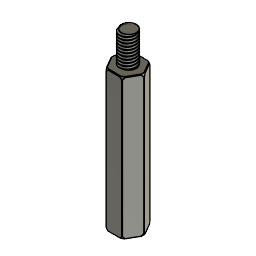
M3 X 25mm Male to Female Brass Spacer (Autodesk Fusion 360 design; units mm, degrees)
Autodesk Fusion 360 part; units mm, degrees
sketch "Sketch1" plane through (0, 0, 0) normal (0, 0, 1) x (1, 0, 0)
  line L0 (-1.4434, 2.5) -> (-2.8868, 0)
  line L1 (-2.8868, 0) -> (-1.4434, -2.5)
  line L2 (-1.4434, -2.5) -> (1.4434, -2.5)
  line L3 (1.4434, -2.5) -> (2.8868, 0)
  line L4 (2.8868, 0) -> (1.4434, 2.5)
  line L5 (1.4434, 2.5) -> (-1.4434, 2.5)
  circle A0 centre (0, 0) radius 1.5
  dimension "d2" = 3
  constraint coincident A0.centre origin
  measures "d2" diameter of A0
extrude "Extrude1" add sketch "Sketch1" along normal blind 25
extrude "Extrude2" add sketch "Sketch1" along normal blind 22.5 from surface at 8 contours A0
thread "Thread1" "ISO Metric profile 3.0 M3x0.5 M3x0.5 6g" major diameter 2.927 minor diameter 2.3555 pitch 0.5 angle 60 modelled right hand crest width 0.0713 on face at (1.4925, -0.1494, 26.8333) crest through (1.4635, 0, 24.875)
thread "Thread2" "ISO Metric profile 3.0 M3x0.5 M3x0.5 6H" major diameter 3.086 minor diameter 2.529 pitch 0.5 angle 60 modelled right hand crest width 0.1368 on face at (1.4925, -0.1494, 2.6667) crest through (1.2645, 0, 0.125)
sketch "Sketch2" plane through (-2.1651, -1.25, 0) normal (-0.866025, -0.5, 0) x (0.5, -0.866025, 0)
  line L0 (-1.4434, 0) -> (1.4434, 0)
  line L1 (1.4434, 0) -> (1.4434, 25)
  line L2 (1.4434, 25) -> (-1.4434, 25)
  line L3 (-1.4434, 25) -> (-1.4434, 0)
  line L4 (-1.4434, 0) -> (-1.4434, 0.5)
  line L5 (-1.4434, 25) -> (-1.4434, 24.5)
  dimension "d12" = 0.5
  dimension "d13" = 0.5
  constraint coincident L0.start L3.end
  constraint perpendicular L0 L4
  constraint coincident L2.end L3.start
  constraint perpendicular L2 L5
  measures "d12" distance of L0.start L4.end
  measures "d13" distance of L2.end L5.end
sketch "Sketch3" plane through (0, 0, 25) normal (0, 0, 1) x (-1, 0, 0)
  arc A0 (-0.634, -1.319) -> (0.634, -1.319) centre (0, 0) ccw
  spline S0 degree 3 poles (-0.634, -1.319) (-0.7449, -1.2523) (-0.8463, -1.1711) (-1.0222, -0.9858) (-1.0965, -0.8832) (-1.239, -0.6161) (-1.2915, -0.4458) (-1.3263, -0.1013) (-1.3109, 0.0692) (-1.2163, 0.3878) (-1.1406, 0.5335) (-0.941, 0.7816) (-0.821, 0.8831) (-0.6847, 0.9583) knots -0.275362 -0.275362 -0.275362 -0.275362 -0.236706 -0.236706 -0.199015 -0.199015 -0.146206 -0.146206 -0.095434 -0.095434 -0.046698 -0.046698 0 0 0 0
  arc A1 (0.6847, 0.9583) -> (-0.6847, 0.9583) centre (0, 0) ccw
  spline S1 degree 3 poles (0.6847, 0.9583) (0.7781, 0.9068) (0.864, 0.8428) (1.019, 0.6916) (1.0868, 0.6046) (1.2259, 0.367) (1.2801, 0.209) (1.3272, -0.1257) (1.317, -0.2994) (1.2301, -0.6403) (1.1516, -0.8035) (0.9334, -1.097) (0.7937, -1.2229) (0.634, -1.319) knots -0.276632 -0.276632 -0.276632 -0.276632 -0.244511 -0.244511 -0.211432 -0.211432 -0.161639 -0.161639 -0.109803 -0.109803 -0.055923 -0.055923 0 0 0 0
  line L0 (-1.4434, -2.5) -> (1.4434, -2.5)
  line L1 (1.4434, -2.5) -> (2.8868, 0)
  line L2 (2.8868, 0) -> (1.4434, 2.5)
  line L3 (1.4434, 2.5) -> (-1.4434, 2.5)
  line L4 (-1.4434, 2.5) -> (-2.8868, 0)
  line L5 (-2.8868, 0) -> (-1.4434, -2.5)
  line L6 (2.8868, 0) -> (2.6368, 0.433)
  line L7 (2.8868, 0) -> (2.6368, -0.433)
  dimension "d14" = 0.5
  dimension "d15" = 0.5
  constraint coincident L1.end L2.start
  constraint parallel L2 L6
  constraint parallel L1 L7
  measures "d14" distance of L1.end L6.end
  measures "d15" distance of L1.end L7.end
sketch "Sketch4" plane through (0, 0, 0) normal (0, 0, -1) x (1, 0, 0)
  spline S0 degree 3 poles (-0.3985, -1.4906) (-0.5834, -1.4231) (-0.7535, -1.3207) (-1.0389, -1.0601) (-1.1532, -0.9065) (-1.3124, -0.5696) (-1.3581, -0.3908) (-1.3767, -0.0326) (-1.352, 0.1432) (-1.259, 0.4082) (-1.2125, 0.5028) (-1.099, 0.6765) (-1.033, 0.7553) (-0.9581, 0.8252) knots 0 0 0 0 0.059039 0.059039 0.116033 0.116033 0.170983 0.170983 0.223888 0.223888 0.255505 0.255505 0.286347 0.286347 0.286347 0.286347
  arc A0 (0.9581, 0.8252) -> (-0.9581, 0.8252) centre (0, 0) ccw
  spline S1 degree 3 poles (0.9581, 0.8252) (1.0802, 0.7112) (1.1784, 0.574) (1.3207, 0.264) (1.3611, 0.093) (1.3757, -0.2618) (1.3471, -0.4423) (1.2212, -0.7891) (1.1226, -0.9512) (0.9156, -1.1792) (0.8244, -1.2577) (0.6232, -1.3929) (0.5136, -1.4486) (0.3985, -1.4906) knots 0 0 0 0 0.050111 0.050111 0.102261 0.102261 0.15645 0.15645 0.212677 0.212677 0.24852 0.24852 0.285143 0.285143 0.285143 0.285143
  arc A1 (-0.3985, -1.4906) -> (0.3985, -1.4906) centre (0, 0) ccw
  line L0 (-1.4434, -2.5) -> (1.4434, -2.5)
  line L1 (1.4434, -2.5) -> (2.8868, 0)
  line L2 (2.8868, 0) -> (1.4434, 2.5)
  line L3 (1.4434, 2.5) -> (-1.4434, 2.5)
  line L4 (-1.4434, 2.5) -> (-2.8868, 0)
  line L5 (-2.8868, 0) -> (-1.4434, -2.5)
  line L6 (-2.8868, 0) -> (-2.6368, 0.433)
  line L7 (-2.8868, 0) -> (-2.6368, -0.433)
  dimension "d16" = 0.5
  dimension "d17" = 0.5
  constraint coincident L4.end L5.start
  constraint parallel L4 L6
  constraint parallel L5 L7
  measures "d16" distance of L4.end L6.end
  measures "d17" distance of L4.end L7.end
ref_plane "WorkPlane1" through (-2.6368, 0.433, 25) normal (0.894427, 0, -0.447214) x (-0.447214, 0, -0.894427)
ref_plane "WorkPlane2" through (-2.6368, 0.433, 0) normal (0.894427, 0, 0.447214) x (0.447214, 0, -0.894427)
sketch "Sketch5" plane through (-2.1094, 0, -1.0547) normal (0.894427, 0, 0.447214) x (0.447214, 0, -0.894427)
  line L0 (-1.8, -0.5) -> (-1.1, -0.5)
  line L1 (-1.1, -0.5) -> (-1.1, 0.5)
  line L2 (-1.1, 0.5) -> (-1.8, 0.5)
  line L3 (-1.8, 0.5) -> (-1.8, -0.5)
  constraint horizontal L0
  constraint vertical L1
  constraint horizontal L2
  constraint vertical L3
extrude "Extrude3" cut sketch "Sketch5" against normal blind 5
sketch "Sketch6" plane through (-12.1094, 0, 6.0547) normal (0.894427, 0, -0.447214) x (-0.447214, 0, -0.894427)
  line L0 (-20.6, 0.5) -> (-21.3, 0.5)
  line L1 (-21.3, 0.5) -> (-21.3, -0.5)
  line L2 (-21.3, -0.5) -> (-20.6, -0.5)
  line L3 (-20.6, -0.5) -> (-20.6, 0.5)
  constraint horizontal L0
  constraint vertical L1
  constraint horizontal L2
  constraint vertical L3
extrude "Extrude4" cut sketch "Sketch6" against normal blind 5
pattern_circular "C-Pattern1" count 6 over 360 about axis through (0, 0, 1.75) along (0, 0, 1) of 2 faces at (-2.7201, 0, 24.8333) (-2.7201, 0, 0.1667)
fillet "Fillet1" radius 0.1 18 edges at (1.4434, -2.5, 12.5) (-1.4434, -2.5, 12.5) (2.8868, 0, 12.5) (1.4434, 2.5, 12.5) (-1.4434, 2.5, 12.5) (-2.8868, 0, 12.5) (-2.1651, 1.25, 25) (0, 2.5, 25) (2.1651, 1.25, 25) (2.1651, -1.25, 25) (0, -2.5, 25) (-2.1651, -1.25, 25) (-2.1651, -1.25, 0) (-2.1651, 1.25, 0) (0, 2.5, 0) (2.1651, 1.25, 0) (2.1651, -1.25, 0) (0, -2.5, 0)
equation "d6 = 25 mm - 8 mm + 5.5 mm"
